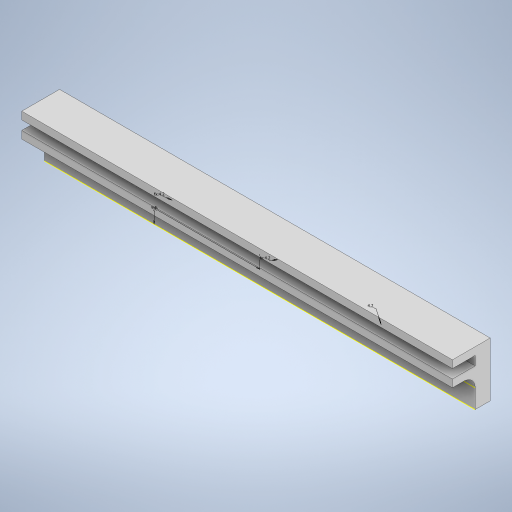
# Autodesk Inventor part: cheeseboard mounts v02
Saved by Autodesk Inventor 2023 (Build 270158000, 158)
## iProperties
Created: 2022-07-11
Part Number: cheeseboard mounts v02
Material: Generic
Document SubType Name: Modeling
Designer: ledap
Density: 1 g/cm^3
Appearance: Default
Author: ledap
Autodesk Inventor part; units mm, degrees
ref_plane "YZ Plane" through (0, 0, 0) normal (1, 0, 0) x (0, 1, 0)
ref_plane "XZ Plane" through (0, 0, 0) normal (0, 1, 0) x (-1, 0, 0)
ref_plane "XY Plane" through (0, 0, 0) normal (0, 0, 1) x (1, 0, 0)
sketch "Sketch1" plane through (0, 0, 0) normal (0, 0, 1) x (1, 0, 0)
  line L0 (142.5, 18) -> (-142.5, 18)
  line L1 (-142.5, 18) -> (-142.5, -18)
  line L2 (-142.5, -18) -> (142.5, -18)
  line L3 (142.5, -18) -> (142.5, 18)
  line L4 (142.5, 18) -> (-142.5, -18) construction
  line L5 (-142.5, 18) -> (142.5, -18) construction
  line L6 (-142.5, 18) -> (142.5, 18)
  line L7 (142.5, 18) -> (142.5, 8)
  line L8 (142.5, 8) -> (-142.5, 8)
  line L9 (-142.5, 8) -> (-142.5, 18)
  point P0 (0, 0)
  point P1 (142.5, 13)
  dimension "d0" = 285
  dimension "d1" = 36
  dimension "d4" = 5
  constraints: 20 end point, 4 parallel, 3 midpoint, 2 horizontal, 2 perpendicular, 1 point on line
  measures "d0" distance of L2.end L1.end
  measures "d1" distance of L1.end L0.end
  measures "d4" distance of L6.end point (142.5, 13)
extrude "Extrusion1" add sketch "Sketch1" along normal blind 10
sketch "Sketch4" plane through (0, 0, 10) normal (0, 0, 1) x (1, 0, 0)
  line L0 (-142.5, 18) -> (-142.5, -18) projected
  line L1 (-142.5, 18) -> (142.5, 18)
  line L2 (142.5, 18) -> (142.5, 13)
  line L3 (142.5, 13) -> (-142.5, 13)
  line L4 (-142.5, 13) -> (-142.5, 18)
  point P0 (0, 0)
  dimension "d5" = 285
  dimension "d6" = 5
  constraints: 8 end point, 2 parallel, 1 horizontal, 1 perpendicular
  measures "d5" distance of L2.end L3.end
  measures "d6" distance of L1.end L2.end
extrude "Extrusion2" add sketch "Sketch4" along normal blind 15
sketch "Sketch5" plane through (0, 0, 10) normal (0, 0, 1) x (1, 0, 0)
  line L0 (-142.5, 18) -> (-142.5, -18) projected
  line L1 (-142.5, 7) -> (142.5, 7)
  line L2 (142.5, 7) -> (142.5, 2)
  line L3 (142.5, 2) -> (-142.5, 2)
  line L4 (-142.5, 2) -> (-142.5, 7)
  line L5 (142.5, 13) -> (-142.5, 13) projected
  point P0 (0, 0)
  dimension "d9" = 285
  dimension "d10" = 5
  dimension "d47" = 11
  constraints: 8 end point, 2 parallel, 1 horizontal, 1 perpendicular, 1 point on line
  measures "d9" distance of L2.end L3.end
  measures "d10" distance of L1.end L2.end
  measures "d47" distance between parallel lines of L3 L5
extrude "Extrusion3" add sketch "Sketch5" along normal blind 15
fillet "Fillet1" radius 7.5 1 edges at (0, 2, 10)
sketch "Sketch6" plane through (0, 0, 10) normal (0, 0, 1) x (1, 0, 0)
  circle A0 centre (-70, -8.5) radius 2.5
  line L0 (-142.5, -5.5) -> (142.5, -5.5) projected
  line L1 (-142.5, -18) -> (142.5, -18) projected
  point P0 (0, 0)
  point P1 (0, -5.5)
  point P2 (0, -5.5)
  dimension "d50" = 70
  dimension "d51" = 9.5
  constraints: 2 midpoint, 1 centre point
  measures "d50" horizontal distance of point (0, 0) A0.centre
  measures "d51" distance from line of L1 A0.centre
hole "Hole1" at (-70, -8.5, 10) direction (0, 0, -1) diameter 5 end through all
sketch "Sketch7" plane through (0, 0, 10) normal (0, 0, 1) x (1, 0, 0)
  circle A0 centre (0, -8.5) radius 2.5
  circle A1 centre (-70, -8.5) radius 2.5 projected
  line L0 (-142.5, -18) -> (142.5, -18) projected
  point P0 (0, 0)
  point P1 (-69.25, -4.8686)
  point P2 (-64.25, -4.8686)
  dimension "d23" = 5
  dimension "d39" = 70
  dimension "d43" = 9.5
  constraints: 1 centre point, 1 other
  measures "d23" diameter of A0
  measures "d39" distance of A0.centre point (-70, -8.5)
  measures "d43" distance from line of L0 A0.centre
hole "Hole2" at (0, -8.5, 10) direction (0, 0, -1) diameter 5 end through all
sketch "Sketch8" plane through (0, 0, 10) normal (0, 0, 1) x (1, 0, 0)
  circle A0 centre (69.4481, -8.5) radius 2.5
  circle A1 centre (0, -8.5) radius 2.5 projected
  line L0 (-142.5, -5.5) -> (142.5, -5.5) projected
  line L1 (-142.5, -18) -> (142.5, -18) projected
  point P0 (0, 0)
  point P1 (-1.3066, -5.3686)
  point P2 (1.3066, -5.3686)
  point P3 (-70, -4.8686)
  dimension "d31" = 5
  dimension "d48" = 7
  constraints: 1 centre point, 2 other
  measures "d31" diameter of A0
  measures "d48" distance edge to line of A0 L1
hole "Hole3" at (69.4481, -8.5, 10) direction (0, 0, -1) diameter 5 end through all
sketch "Sketch11" plane through (0, 0, 0) normal (0, 0, -1) x (-1, 0, 0)
  circle A0 centre (-69.4481, -8.5) radius 2.5 projected
  circle A1 centre (-69.4481, -8.5) radius 2.1
  circle A2 centre (0, -8.5) radius 2.5 projected
  circle A3 centre (0, -8.5) radius 2.1
  circle A4 centre (70, -8.5) radius 2.5 projected
  circle A5 centre (70, -8.5) radius 2.1
  point P0 (0, 0)
  dimension "d52" = 4.2
  dimension "d53" = 4.2
  dimension "d54" = 4.2
  constraints: 3 centre point, 3 coincident
  measures "d52" diameter of A1
  measures "d53" diameter of A3
  measures "d54" diameter of A5
equation "\"d53\" = d52"
equation "\"d54\" = d52"
body "Solid1"
